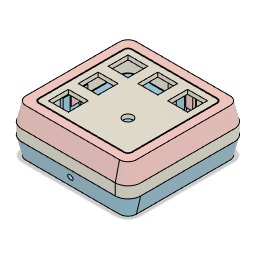
Pico_Macropad v37 (Autodesk Fusion 360 design; units mm, degrees)
Autodesk Fusion 360 part; units mm, degrees
note: some values were not read from the file. Set by a fixed rule: which sketch regions a step uses.
ref_plane "WorkPlane3" through (0, 25.4, 0) normal (0, 1, 0) x (0, 0, 1) in component "switchesPlate"
sketch "keycapsSwitches" plane through (0, 25.4, 0) normal (0, 1, 0) x (1, 0, 0) in component "switchesPlate"
  line L0 (-30.15, -30.15) -> (-12.05, -30.15) construction
  line L1 (-12.05, -30.15) -> (-12.05, -12.05) construction
  line L2 (-12.05, -12.05) -> (-30.15, -12.05) construction
  line L3 (-30.15, -12.05) -> (-30.15, -30.15) construction
  line L4 (-28.1, -28.1) -> (-14.1, -28.1)
  line L5 (-14.1, -28.1) -> (-14.1, -14.1)
  line L6 (-14.1, -14.1) -> (-28.1, -14.1)
  line L7 (-28.1, -14.1) -> (-28.1, -28.1)
  line L8 (-21.1, -12.05) -> (-21.1, -30.15) construction
  line L9 (-12.05, -21.1) -> (-30.15, -21.1) construction
  line L10 (-9.05, -12.05) -> (-9.05, -30.15) construction
  line L11 (7, -28.1) -> (7, -14.1)
  line L12 (-7, -28.1) -> (7, -28.1)
  line L13 (-7, -14.1) -> (-7, -28.1)
  line L14 (9.05, -21.1) -> (-9.05, -21.1) construction
  line L15 (7, -14.1) -> (-7, -14.1)
  line L16 (9.05, -12.05) -> (-9.05, -12.05) construction
  line L17 (0, -12.05) -> (0, -30.15) construction
  line L18 (-9.05, -30.15) -> (9.05, -30.15) construction
  line L19 (9.05, -30.15) -> (9.05, -12.05) construction
  line L20 (12.05, -12.05) -> (12.05, -30.15) construction
  line L21 (30.15, -21.1) -> (12.05, -21.1) construction
  line L22 (12.05, -30.15) -> (30.15, -30.15) construction
  line L23 (28.1, -14.1) -> (14.1, -14.1)
  line L24 (30.15, -12.05) -> (12.05, -12.05) construction
  line L25 (28.1, -28.1) -> (28.1, -14.1)
  line L26 (21.1, -12.05) -> (21.1, -30.15) construction
  line L27 (30.15, -30.15) -> (30.15, -12.05) construction
  line L28 (14.1, -14.1) -> (14.1, -28.1)
  line L29 (14.1, -28.1) -> (28.1, -28.1)
  line L30 (12.05, 9.05) -> (12.05, -9.05) construction
  line L31 (30.15, 0) -> (12.05, 0) construction
  line L32 (12.05, -9.05) -> (30.15, -9.05) construction
  line L33 (30.15, 9.05) -> (12.05, 9.05) construction
  line L34 (21.1, 9.05) -> (21.1, -9.05) construction
  line L35 (28.1, -7) -> (28.1, 7)
  line L36 (28.1, 7) -> (14.1, 7)
  line L37 (14.1, -7) -> (28.1, -7)
  line L38 (30.15, -9.05) -> (30.15, 9.05) construction
  line L39 (14.1, 7) -> (14.1, -7)
  line L40 (21.1, 30.15) -> (21.1, 12.05) construction
  line L41 (30.15, 12.05) -> (30.15, 30.15) construction
  line L42 (14.1, 14.1) -> (28.1, 14.1)
  line L43 (28.1, 28.1) -> (14.1, 28.1)
  line L44 (30.15, 21.1) -> (12.05, 21.1) construction
  line L45 (14.1, 28.1) -> (14.1, 14.1)
  line L46 (30.15, 30.15) -> (12.05, 30.15) construction
  line L47 (12.05, 30.15) -> (12.05, 12.05) construction
  line L48 (28.1, 14.1) -> (28.1, 28.1)
  line L49 (12.05, 12.05) -> (30.15, 12.05) construction
  line L50 (-33.15, 33.15) -> (33.15, 33.15) construction
  line L51 (33.15, 33.15) -> (33.15, -33.15) construction
  line L52 (33.15, -33.15) -> (-33.15, -33.15) construction
  line L53 (-33.15, -33.15) -> (-33.15, 33.15) construction
  dimension "d136" = 18.1
  dimension "d147" = 14
  dimension "d150" = 7
  dimension "d151" = 7
  dimension "d152" = 18.1
  dimension "d153" = 14
  dimension "d154" = 7
  dimension "d155" = 7
  dimension "d156" = 18.1
  dimension "d157" = 14
  dimension "d158" = 7
  dimension "d159" = 7
  dimension "d160" = 18.1
  dimension "d161" = 14
  dimension "d162" = 7
  dimension "d163" = 7
  dimension "d164" = 18.1
  dimension "d165" = 14
  dimension "d166" = 7
  dimension "d167" = 7
  dimension "d168" = 3
  dimension "d169" = 3
  dimension "d170" = 3
  dimension "d171" = 3
  dimension "d173" = 3
  dimension "d174" = 3
  dimension "d175" = 3
  dimension "d176" = 3
  constraint horizontal L0
  constraint vertical L1
  constraint horizontal L2
  constraint vertical L3
  constraint equal L1 L2
  constraint horizontal L4
  constraint vertical L5
  constraint horizontal L6
  constraint vertical L7
  constraint equal L4 L5
  constraint midpoint L2 L8.start
  constraint midpoint L0 L8.end
  constraint midpoint L1 L9.start
  constraint midpoint L3 L9.end
  constraint horizontal L18
  constraint vertical L19
  constraint horizontal L16
  constraint vertical L10
  constraint equal L16 L19
  constraint horizontal L12
  constraint vertical L11
  constraint horizontal L15
  constraint vertical L13
  constraint equal L11 L12
  constraint midpoint L17.start L16
  constraint midpoint L17.end L18
  constraint midpoint L14.start L19
  constraint midpoint L14.end L10
  constraint horizontal L22
  constraint vertical L27
  constraint horizontal L24
  constraint vertical L20
  constraint equal L24 L27
  constraint horizontal L29
  constraint vertical L25
  constraint horizontal L23
  constraint vertical L28
  constraint equal L25 L29
  constraint midpoint L26.start L24
  constraint midpoint L26.end L22
  constraint midpoint L21.start L27
  constraint midpoint L21.end L20
  constraint horizontal L32
  constraint vertical L38
  constraint horizontal L33
  constraint vertical L30
  constraint equal L33 L38
  constraint horizontal L37
  constraint vertical L35
  constraint horizontal L36
  constraint vertical L39
  constraint equal L35 L37
  constraint midpoint L34.start L33
  constraint midpoint L34.end L32
  constraint midpoint L31.start L38
  constraint midpoint L31.end L30
  constraint horizontal L49
  constraint vertical L41
  constraint horizontal L46
  constraint vertical L47
  constraint equal L41 L46
  constraint horizontal L42
  constraint vertical L48
  constraint horizontal L43
  constraint vertical L45
  constraint equal L42 L48
  constraint midpoint L40.start L46
  constraint midpoint L40.end L49
  constraint midpoint L44.start L41
  constraint midpoint L44.end L47
  constraint coincident L20 L30.end
  constraint coincident L30 L47.end
  constraint coincident origin L17
  constraint coincident L5.end L15
  constraint coincident L18 L20.end
  constraint coincident origin L31
  constraint horizontal L50
  constraint vertical L51
  constraint horizontal L52
  constraint vertical L53
  measures "d136" distance of L1.end L2.end
  measures "d147" distance of L4.end L5.end
  measures "d150" distance of L5.end L8
  measures "d151" distance of L4.end L9
  measures "d152" distance of L16.start L10.start
  measures "d153" distance of L11.start L11.end
  measures "d154" distance of L11.end L17
  measures "d155" distance of L11.start L14
  measures "d156" distance of L20.start L24.start
  measures "d157" distance of L23.start L25.start
  measures "d158" distance of L23.start L26
  measures "d159" distance of L25.start L21
  measures "d160" distance of L30.start L33.start
  measures "d161" distance of L35.end L35.start
  measures "d162" distance of L35.end L34
  measures "d163" distance of L35.start L31
  measures "d164" distance of L46.end L41.end
  measures "d165" distance of L43.start L42.end
  measures "d166" distance of L43.start L40
  measures "d167" distance of L42.end L44
  measures "d168" horizontal distance of L1.end L10.start
  measures "d169" distance of L16.start L20.start
  measures "d170" distance of L24.start L32.end
  measures "d171" distance of L33.start L41.start
  measures "d173" distance of L22.end L52
  measures "d174" distance of L41.end L51
  measures "d175" distance of L41.end L50
  measures "d176" distance of L3 L52.end
sketch "encoder" plane through (0, 25.4, 0) normal (0, 1, 0) x (1, 0, 0) in component "switchesPlate"
  line L0 (12.05, 30.15) -> (12.05, 12.05)
  line L1 (12.05, 9.05) -> (12.05, -9.05)
  line L2 (9.05, -12.05) -> (-9.05, -12.05)
  line L3 (-12.05, -12.05) -> (-30.15, -12.05)
  line L4 (-33.15, 33.15) -> (33.15, 33.15)
  line L5 (-33.15, -33.15) -> (-33.15, 33.15)
  line L6 (12.05, -12.05) -> (-33.15, 33.15) construction
  circle A0 centre (-10.55, 10.55) radius 3.5
  dimension "d177" = 7
  constraint coincident L4.start L5.end
  constraint coincident L2 L6.start
  constraint coincident L1 L6.start
  constraint midpoint L6 A0.centre
  measures "d177" diameter of A0
ref_plane "WorkPlane4" through (0, 22.4, 0) normal (0, 1, 0) x (0, 0, 1) in component "switchesPlate"
sketch "switchPlate" plane through (0, 22.4, 0) normal (0, 1, 0) x (1, 0, 0) in component "switchesPlate"
  line L0 (-36.15, 36.15) -> (36.15, 36.15)
  line L1 (36.15, 36.15) -> (36.15, -36.15)
  line L2 (36.15, -36.15) -> (-36.15, -36.15)
  line L3 (-36.15, -36.15) -> (-36.15, 36.15)
  line L4 (-33.15, 33.15) -> (33.15, 33.15)
  line L5 (33.15, 33.15) -> (33.15, -33.15)
  line L6 (33.15, -33.15) -> (-33.15, -33.15)
  line L7 (-33.15, -33.15) -> (-33.15, 33.15)
  line L8 (-33.15, 33.15) -> (33.15, 33.15)
  point P0 (33.15, -33.15)
  point P1 (-33.15, 33.15)
  point P2 (33.15, 33.15)
  point P3 (33.15, 33.15)
  dimension "d180" = 3
  dimension "d181" = 3
  dimension "d182" = 3
  dimension "d183" = 3
  constraint horizontal L0
  constraint vertical L1
  constraint horizontal L2
  constraint vertical L3
  constraint horizontal L4
  constraint vertical L5
  constraint horizontal L6
  constraint vertical L7
  constraint coincident P0 L5.end
  constraint coincident P1 L4.start
  measures "d180" horizontal distance of L0.end P3
  measures "d181" horizontal distance of L0.start L4.start
  measures "d182" vertical distance of L1.end P0
  measures "d183" vertical distance of L0.end P3
extrude "Extrude13" add sketch "switchPlate" along normal blind 1 contours L0 L1 L2 L3 | L4 L5 L6 L7 L8 makes body 1 in component "switchesPlate"
extrude "Extrude14" add sketch "switchPlate" along normal blind 3 contours L4 L5 L6 L7 L8 bodies 1 in component "switchesPlate"
fillet "Fillet4" radius 3 8 edges at (33.15, 24.4, 33.15) (36.15, 22.9, 36.15) (36.15, 22.9, -36.15) (33.15, 24.4, -33.15) (-33.15, 24.4, -33.15) (-36.15, 22.9, -36.15) (-36.15, 22.9, 36.15) (-33.15, 24.4, 33.15) on bodies 1 in component "switchesPlate"
sketch "loftIn1" plane through (0, 25.4, 0) normal (0, 1, 0) x (-1, 0, 0) in component "case"
  arc A0 (33.15, 30.15) -> (30.15, 33.15) centre (30.15, 30.15) ccw
  line L0 (30.15, 33.15) -> (-30.15, 33.15)
  arc A1 (-30.15, 33.15) -> (-33.15, 30.15) centre (-30.15, 30.15) ccw
  line L1 (-33.15, 30.15) -> (-33.15, -30.15)
  arc A2 (-33.15, -30.15) -> (-30.15, -33.15) centre (-30.15, -30.15) ccw
  line L2 (-30.15, -33.15) -> (30.15, -33.15)
  arc A3 (30.15, -33.15) -> (33.15, -30.15) centre (30.15, -30.15) ccw
  line L3 (33.15, -30.15) -> (33.15, 30.15)
  arc A4 (36.15, 33.15) -> (33.15, 36.15) centre (33.15, 33.15) ccw
  line L4 (-33.15, 36.15) -> (33.15, 36.15)
  line L5 (36.15, 33.15) -> (36.15, -33.15)
  arc A5 (33.15, -36.15) -> (36.15, -33.15) centre (33.15, -33.15) ccw
  line L6 (33.15, -36.15) -> (-33.15, -36.15)
  arc A6 (-36.15, -33.15) -> (-33.15, -36.15) centre (-33.15, -33.15) ccw
  line L7 (-36.15, -33.15) -> (-36.15, 33.15)
  arc A7 (-33.15, 36.15) -> (-36.15, 33.15) centre (-33.15, 33.15) ccw
  line L8 (33.15, -39.15) -> (-33.15, -39.15)
  arc A8 (-39.15, -33.15) -> (-33.15, -39.15) centre (-33.15, -33.15) ccw
  line L9 (-39.15, -33.15) -> (-39.15, 33.15)
  arc A9 (-33.15, 39.15) -> (-39.15, 33.15) centre (-33.15, 33.15) ccw
  line L10 (-33.15, 39.15) -> (33.15, 39.15)
  arc A10 (39.15, 33.15) -> (33.15, 39.15) centre (33.15, 33.15) ccw
  line L11 (39.15, 33.15) -> (39.15, -33.15)
  arc A11 (33.15, -39.15) -> (39.15, -33.15) centre (33.15, -33.15) ccw
  dimension "d190" = 3
ref_plane "WorkPlane4" through (0, 12.7, 0) normal (0, 1, 0) x (0, 0, 1) in component "case"
sketch "loftin2" plane through (0, 12.7, 0) normal (0, 1, 0) x (1, 0, 0) in component "case"
  arc A0 (33.15, -39.15) -> (39.15, -33.15) centre (33.15, -33.15) ccw
  line L0 (33.15, -39.15) -> (-33.15, -39.15)
  arc A1 (-39.15, -33.15) -> (-33.15, -39.15) centre (-33.15, -33.15) ccw
  line L1 (-39.15, -33.15) -> (-39.15, 33.15)
  arc A2 (-33.15, 39.15) -> (-39.15, 33.15) centre (-33.15, 33.15) ccw
  line L2 (-33.15, 39.15) -> (33.15, 39.15)
  arc A3 (39.15, 33.15) -> (33.15, 39.15) centre (33.15, 33.15) ccw
  line L3 (39.15, 33.15) -> (39.15, -33.15)
  arc A4 (-42.15, -33.15) -> (-33.15, -42.15) centre (-33.15, -33.15) ccw
  line L4 (33.15, -42.15) -> (-33.15, -42.15)
  arc A5 (33.15, -42.15) -> (42.15, -33.15) centre (33.15, -33.15) ccw
  line L5 (42.15, 33.15) -> (42.15, -33.15)
  arc A6 (42.15, 33.15) -> (33.15, 42.15) centre (33.15, 33.15) ccw
  line L6 (-33.15, 42.15) -> (33.15, 42.15)
  arc A7 (-33.15, 42.15) -> (-42.15, 33.15) centre (-33.15, 33.15) ccw
  line L7 (-42.15, -33.15) -> (-42.15, 33.15)
  dimension "d192" = 3
loft "Loft8" add profiles "loftin2" section 1 face at (11.05, 22.4, -12.05) section 2 contours A0 L0 A1 L1 A2 L2 A3 L3 separate body on bodies 1 makes body 2 in component "case"
loft "Loft9" add profiles "loftin2", "loftIn1" section 1 section 2 contours L8 A8 L9 A9 L10 A10 L11 A11 separate body makes body 3 in component "case"
combine "Combine9" operation cut target body 3 tool bodies 2 keep tools in component "case"
sketch "tooth" plane through (0, 0, 0) normal (0, 0, 1) x (1, 0, 0) in component "case"
  line L0 (39.15, 25.4) -> (-39.15, 25.4)
  line L1 (42.15, 12.7) -> (39.15, 12.7)
  line L2 (-39.15, 12.7) -> (-42.15, 12.7)
  line L3 (42.15, 12.7) -> (39.15, 25.4)
  line L4 (-42.15, 12.7) -> (-39.15, 25.4)
  line L5 (39.15, 12.7) -> (-39.15, 12.7)
  line L6 (36.15, 22.4) -> (-36.15, 22.4)
  line L7 (36.15, 22.4) -> (39.15, 12.7)
  line L8 (-36.15, 22.4) -> (-39.15, 12.7)
  line L9 (-39.15, 12.7) -> (-39.15, 4.7)
  line L10 (-39.15, 4.7) -> (-37.15, 4.7)
  line L11 (-37.15, 4.7) -> (-37.15, 19.1667)
  line L12 (-37.15, 19.1667) -> (-39.15, 12.7)
  dimension "d221" = 2
  dimension "d222" = 8
  constraint coincident L2.start L5.end
  constraint perpendicular L2 L9
  constraint perpendicular L9 L10
  constraint perpendicular L5 L11
  constraint coincident L8 L11.end
  constraint coincident L11.end L12.start
  measures "d221" distance of L9.end L10.end
  measures "d222" distance of L2.start L9.end
extrude "Extrude3" add sketch "tooth" along normal mid plane 6 contours L5 L8 L11 L12 | L5 L9 L10 L11 bodies 3 in component "case"
pattern_circular "C-Pattern1" count 2 over 360 about axis through (0, 1.75, 0) along (0, 1, 0) of "Extrude3" in component "case"
ref_plane "WorkPlane5" through (3.75, 0, 0) normal (1, 0, 0) x (0, 1, 0) in component "case"
sketch "doubletooth" plane through (3.75, 0, 0) normal (1, 0, 0) x (0, 0, -1) in component "case"
  line L0 (-42.15, 12.7) -> (42.15, 12.7)
  line L1 (-42.15, 12.7) -> (-39.15, 25.4)
  line L2 (-39.15, 25.4) -> (39.15, 25.4)
  line L3 (-3, 4.7) -> (3, 4.7)
  line L4 (3, 4.7) -> (3, 12.7)
  line L5 (-3, 12.7) -> (3, 12.7)
  line L6 (-3, 12.7) -> (-3, 4.7)
  line L7 (3, 12.7) -> (3, 19.1667)
  line L8 (3, 19.1667) -> (-3, 19.1667)
  line L9 (-3, 19.1667) -> (-3, 12.7)
  line L10 (-39.15, 12.7) -> (-3, 12.7)
  line L11 (-39.15, 12.7) -> (-36.15, 22.4)
  line L12 (-36.15, 22.4) -> (36.15, 22.4)
  line L13 (-3, 12.7) -> (-39.15, 12.7)
  line L14 (-3, 12.7) -> (-3, 19.1667)
  line L15 (-3, 19.1667) -> (3, 19.1667)
  line L16 (3, 19.1667) -> (3, 12.7)
  line L17 (3, 12.7) -> (39.15, 12.7)
  line L18 (-37.15, 19.1667) -> (-37.15, 4.7)
  line L19 (-37.15, 4.7) -> (-39.15, 4.7)
  line L20 (-39.15, 4.7) -> (-39.15, 12.7)
  line L21 (-39.15, 25.4) -> (-42.15, 12.7)
  line L22 (-36.15, 22.4) -> (-39.15, 12.7)
  dimension "d230" = 2
  constraint perpendicular L10 L18
  constraint coincident L10.start L11.start
  constraint coincident L3 L19.end
  constraint perpendicular L18 L19
  constraint perpendicular L19 L20
  constraint coincident L11.end L12.start
  constraint coincident L11 L18.start
  measures "d230" distance of L18.end L19.end
extrude "Extrude6" add sketch "doubletooth" along normal blind 5 contours L0 L10 L11 L13 L18 L22 | L0 L10 L13 L18 L19 L20 bodies 3 in component "case"
mirror "Mirror4" about plane through (0, 0, 0) normal (1, 0, 0) of "Extrude6" in component "case"
mirror "Mirror5" about plane through (0, 0, 0) normal (0, 0, 1) of "Extrude6", "Mirror4" in component "case"
sketch "bandSketch" plane through (0, 12.7, 0) normal (0, -1, 0) x (1, 0, 0) in component "case"
  line L0 (-39.15, -3) -> (-39.15, 3)
  spline S0 degree 3 poles (33.15, 42.15) (34.1498, 42.15) (35.3159, 41.9726) (36.4656, 41.517) (37.3209, 41.1781) (38.1632, 40.6875) (38.9102, 40.0652) (40.0083, 39.1505) (40.8849, 37.9488) (41.422, 36.696) (41.9461, 35.4734) (42.15, 34.2167) (42.15, 33.15) (42.15, 11.05) (42.15, -11.05) (42.15, -33.15) (42.15, -34.1498) (41.9726, -35.3159) (41.517, -36.4656) (41.1781, -37.3209) (40.6875, -38.1632) (40.0652, -38.9102) (39.1505, -40.0083) (37.9488, -40.8849) (36.696, -41.422) (35.4734, -41.9461) (34.2167, -42.15) (33.15, -42.15) (11.05, -42.15) (-11.05, -42.15) (-33.15, -42.15) (-34.1498, -42.15) (-35.3159, -41.9726) (-36.4656, -41.517) (-37.3209, -41.1781) (-38.1632, -40.6875) (-38.9102, -40.0652) (-40.0083, -39.1505) (-40.8849, -37.9488) (-41.422, -36.696) (-41.9461, -35.4734) (-42.15, -34.2167) (-42.15, -33.15) (-42.15, -11.05) (-42.15, 11.05) (-42.15, 33.15) (-42.15, 34.1498) (-41.9726, 35.3159) (-41.517, 36.4656) (-41.1781, 37.3209) (-40.6875, 38.1632) (-40.0652, 38.9102) (-39.1505, 40.0083) (-37.9488, 40.8849) (-36.696, 41.422) (-35.4734, 41.9461) (-34.2167, 42.15) (-33.15, 42.15) (-11.05, 42.15) (11.05, 42.15) (33.15, 42.15) knots 0 0 0 0 0.009612 0.009612 0.009612 0.016762 0.016762 0.016762 0.027271 0.027271 0.027271 0.037527 0.037527 0.037527 0.25 0.25 0.25 0.259612 0.259612 0.259612 0.266762 0.266762 0.266762 0.277271 0.277271 0.277271 0.287527 0.287527 0.287527 0.5 0.5 0.5 0.509612 0.509612 0.509612 0.516762 0.516762 0.516762 0.527271 0.527271 0.527271 0.537527 0.537527 0.537527 0.75 0.75 0.75 0.759612 0.759612 0.759612 0.766762 0.766762 0.766762 0.777271 0.777271 0.777271 0.787527 0.787527 0.787527 1 1 1 1
  line L1 (-33.15, 39.15) -> (-8.75, 39.15)
  line L2 (39.15, 3) -> (39.15, -3)
  line L3 (-8.75, 39.15) -> (-3.75, 39.15)
  line L4 (-3.75, 39.15) -> (3.75, 39.15)
  line L5 (3.75, 39.15) -> (8.75, 39.15)
  spline S1 degree 3 poles (8.75, 39.15) (16.8833, 39.15) (25.0167, 39.15) (33.15, 39.15) (33.7471, 39.15) (34.5104, 39.053) (35.2899, 38.7554) (35.8698, 38.534) (36.4549, 38.2028) (36.9737, 37.7738) (37.7361, 37.1433) (38.3397, 36.2995) (38.6931, 35.4465) (39.038, 34.6141) (39.15, 33.787) (39.15, 33.15) (39.15, 23.1) (39.15, 13.05) (39.15, 3) knots 0.14292 0.14292 0.14292 0.14292 0.226147 0.226147 0.226147 0.232257 0.232257 0.232257 0.236802 0.236802 0.236802 0.243482 0.243482 0.243482 0.25 0.25 0.25 0.352841 0.352841 0.352841 0.352841
  spline S2 degree 3 poles (39.15, -3) (39.15, -13.05) (39.15, -23.1) (39.15, -33.15) (39.15, -33.7471) (39.053, -34.5104) (38.7554, -35.2899) (38.534, -35.8698) (38.2028, -36.4549) (37.7738, -36.9737) (37.1433, -37.7361) (36.2995, -38.3397) (35.4465, -38.6931) (34.6141, -39.038) (33.787, -39.15) (33.15, -39.15) (25.0167, -39.15) (16.8833, -39.15) (8.75, -39.15) knots 0.373307 0.373307 0.373307 0.373307 0.476147 0.476147 0.476147 0.482257 0.482257 0.482257 0.486802 0.486802 0.486802 0.493482 0.493482 0.493482 0.5 0.5 0.5 0.583228 0.583228 0.583228 0.583228
  line L6 (8.75, -39.15) -> (3.75, -39.15)
  line L7 (3.75, -39.15) -> (-3.75, -39.15)
  line L8 (-3.75, -39.15) -> (-8.75, -39.15)
  spline S3 degree 3 poles (-8.75, -39.15) (-16.8833, -39.15) (-25.0167, -39.15) (-33.15, -39.15) (-33.7471, -39.15) (-34.5104, -39.053) (-35.2899, -38.7554) (-35.8698, -38.534) (-36.4549, -38.2028) (-36.9737, -37.7738) (-37.7361, -37.1433) (-38.3397, -36.2995) (-38.6931, -35.4465) (-39.038, -34.6141) (-39.15, -33.787) (-39.15, -33.15) (-39.15, -23.1) (-39.15, -13.05) (-39.15, -3) knots 0.64292 0.64292 0.64292 0.64292 0.726147 0.726147 0.726147 0.732257 0.732257 0.732257 0.736802 0.736802 0.736802 0.743482 0.743482 0.743482 0.75 0.75 0.75 0.852841 0.852841 0.852841 0.852841
  spline S4 degree 3 poles (-39.15, 3) (-39.15, 13.05) (-39.15, 23.1) (-39.15, 33.15) (-39.15, 33.7471) (-39.053, 34.5104) (-38.7554, 35.2899) (-38.534, 35.8698) (-38.2028, 36.4549) (-37.7738, 36.9737) (-37.1433, 37.7361) (-36.2995, 38.3397) (-35.4465, 38.6931) (-34.6141, 39.038) (-33.787, 39.15) (-33.15, 39.15) knots 0.873307 0.873307 0.873307 0.873307 0.976147 0.976147 0.976147 0.982257 0.982257 0.982257 0.986802 0.986802 0.986802 0.993482 0.993482 0.993482 1 1 1 1
extrude "Extrude4" add sketch "bandSketch" along normal up to surface (8 mm away) separate body makes body 4 in component "case"
copy_body "CopyPasteBodies1" bodies 3 makes body 5
move_body "Move1" bodies 5 to x (0, 0, 1) y (0, -1, 0) z (1, 0, 0) at (0, 22.4, 0)
copy_body "CutPasteBodies4" bodies 5 removing the originals makes body 6 in component "case"
combine "Combine10" operation cut target body 3 tool bodies 1 keep tools in component "case"
extrude "Extrude15" cut sketch "encoder" sketch "keycapsSwitches" along normal up to surface of sketch 2 end surface through (0, 22.4, 0) normal (0, -1, 0) offset 0 bodies 1 in component "switchesPlate"
sketch "tolerancePlateTop" plane through (0, 25.4, 0) normal (0, 1, 0) x (-1, 0, 0) in component "switchesPlate"
  line L0 (-14.1, 28.1) -> (-14.1, 14.1)
  line L1 (-14.1, 14.1) -> (-28.1, 14.1)
  line L2 (-28.1, 14.1) -> (-28.1, 28.1)
  line L3 (-28.1, 28.1) -> (-14.1, 28.1)
  line L4 (-14.1, -7) -> (-28.1, -7)
  line L5 (-28.1, -7) -> (-28.1, 7)
  line L6 (-28.1, 7) -> (-14.1, 7)
  line L7 (-14.1, 7) -> (-14.1, -7)
  circle A0 centre (10.55, -10.55) radius 3.5
  line L8 (-7, 14.1) -> (-7, 28.1)
  line L9 (-7, 28.1) -> (7, 28.1)
  line L10 (7, 28.1) -> (7, 14.1)
  line L11 (7, 14.1) -> (-7, 14.1)
  line L12 (-28.1, -14.1) -> (-14.1, -14.1)
  line L13 (-14.1, -14.1) -> (-14.1, -28.1)
  line L14 (-14.1, -28.1) -> (-28.1, -28.1)
  line L15 (-28.1, -28.1) -> (-28.1, -14.1)
  line L16 (28.1, 14.1) -> (14.1, 14.1)
  line L17 (14.1, 14.1) -> (14.1, 28.1)
  line L18 (14.1, 28.1) -> (28.1, 28.1)
  line L19 (28.1, 28.1) -> (28.1, 14.1)
  arc A1 (33.15, 30.15) -> (30.15, 33.15) centre (30.15, 30.15) ccw
  line L20 (30.15, 33.15) -> (-30.15, 33.15)
  arc A2 (-30.15, 33.15) -> (-33.15, 30.15) centre (-30.15, 30.15) ccw
  line L21 (-33.15, 30.15) -> (-33.15, -30.15)
  arc A3 (-33.15, -30.15) -> (-30.15, -33.15) centre (-30.15, -30.15) ccw
  line L22 (-30.15, -33.15) -> (30.15, -33.15)
  arc A4 (30.15, -33.15) -> (33.15, -30.15) centre (30.15, -30.15) ccw
  line L23 (33.15, -30.15) -> (33.15, 30.15)
  line L24 (30.15, 32.65) -> (-30.15, 32.65)
  arc A5 (-30.15, 32.65) -> (-32.65, 30.15) centre (-30.15, 30.15) ccw
  line L25 (-32.65, 30.15) -> (-32.65, -30.15)
  arc A6 (-32.65, -30.15) -> (-30.15, -32.65) centre (-30.15, -30.15) ccw
  line L26 (-30.15, -32.65) -> (30.15, -32.65)
  arc A7 (30.15, -32.65) -> (32.65, -30.15) centre (30.15, -30.15) ccw
  line L27 (32.65, -30.15) -> (32.65, 30.15)
  arc A8 (32.65, 30.15) -> (30.15, 32.65) centre (30.15, 30.15) ccw
  dimension "d208" = -0.5
extrude "Extrude16" cut sketch "tolerancePlateTop" against normal up to surface (2 mm away) contours A1 L20 A2 L21 A3 L22 A4 L23 bodies 1 in component "switchesPlate"
sketch "tolerancePlateInner" plane through (0, 23.4, 0) normal (0, 1, 0) x (-1, 0, 0) in component "switchesPlate"
  arc A0 (36.15, 33.15) -> (33.15, 36.15) centre (33.15, 33.15) ccw
  line L0 (33.15, 36.15) -> (-33.15, 36.15)
  arc A1 (-33.15, 36.15) -> (-36.15, 33.15) centre (-33.15, 33.15) ccw
  line L1 (-36.15, 33.15) -> (-36.15, -33.15)
  arc A2 (-36.15, -33.15) -> (-33.15, -36.15) centre (-33.15, -33.15) ccw
  line L2 (-33.15, -36.15) -> (33.15, -36.15)
  arc A3 (33.15, -36.15) -> (36.15, -33.15) centre (33.15, -33.15) ccw
  line L3 (36.15, -33.15) -> (36.15, 33.15)
  arc A4 (33.15, -35.65) -> (35.65, -33.15) centre (33.15, -33.15) ccw
  line L4 (35.65, -33.15) -> (35.65, 33.15)
  arc A5 (35.65, 33.15) -> (33.15, 35.65) centre (33.15, 33.15) ccw
  line L5 (33.15, 35.65) -> (-33.15, 35.65)
  arc A6 (-33.15, 35.65) -> (-35.65, 33.15) centre (-33.15, 33.15) ccw
  line L6 (-35.65, 33.15) -> (-35.65, -33.15)
  arc A7 (-35.65, -33.15) -> (-33.15, -35.65) centre (-33.15, -33.15) ccw
  line L7 (-33.15, -35.65) -> (33.15, -35.65)
  line L8 (32.65, 30.15) -> (32.65, -30.15)
  arc A8 (30.15, -32.65) -> (32.65, -30.15) centre (30.15, -30.15) ccw
  line L9 (30.15, -32.65) -> (-30.15, -32.65)
  arc A9 (-32.65, -30.15) -> (-30.15, -32.65) centre (-30.15, -30.15) ccw
  line L10 (-32.65, -30.15) -> (-32.65, 30.15)
  arc A10 (-30.15, 32.65) -> (-32.65, 30.15) centre (-30.15, 30.15) ccw
  line L11 (-30.15, 32.65) -> (30.15, 32.65)
  arc A11 (32.65, 30.15) -> (30.15, 32.65) centre (30.15, 30.15) ccw
  dimension "d211" = -0.5
extrude "Extrude17" cut sketch "tolerancePlateInner" against normal up to surface (1 mm away) contours A0 L0 A1 L1 A2 L2 A3 L3 bodies 1 in component "switchesPlate"
move_body "Move5" bodies 6 to x (1, 0, 0) y (0, 1, 0) z (0, 0, 1) at (0, -5, 0) in component "case"
sketch "USBhole" plane through (0, 0, 0) normal (0, 0, 1) x (1, 0, 0) in component "case"
  line L0 (-3, 12.7) -> (3, 12.7)
  line L1 (3, 4.7) -> (3, 12.7)
  line L2 (-39.15, -8) -> (39.15, -8)
  line L3 (-42.15, 4.7) -> (-39.15, 4.7)
  line L4 (-37.15, 4.7) -> (-3, 4.7)
  line L5 (3, 4.7) -> (37.15, 4.7)
  line L6 (39.15, 4.7) -> (42.15, 4.7)
  line L7 (-42.15, 4.7) -> (-39.15, -8)
  line L8 (42.15, 4.7) -> (39.15, -8)
  circle A0 centre (0, -1.1) radius 1.9
  line L9 (0, 1.75) -> (0, 22.5)
  line L10 (-1.9, 0.8) -> (1.9, 0.8) construction
  line L11 (1.9, 0.8) -> (1.9, -3) construction
  line L12 (1.9, -3) -> (-1.9, -3) construction
  line L13 (-1.9, -3) -> (-1.9, 0.8) construction
  line L14 (-39.15, 4.7) -> (-39.15, 12.7)
  line L15 (-37.15, 12.7) -> (-37.15, 4.7)
  line L16 (-39.15, 12.7) -> (-37.15, 12.7)
  line L17 (39.15, 4.7) -> (39.15, 12.7)
  line L18 (37.15, 12.7) -> (37.15, 4.7)
  line L19 (39.15, 12.7) -> (37.15, 12.7)
  line L20 (-3, 12.7) -> (-3, 4.7)
  line L21 (36.15, -5) -> (-36.15, -5)
  dimension "d216" = 3.8
  dimension "d231" = 2
  constraint horizontal L10
  constraint vertical L11
  constraint horizontal L12
  constraint vertical L13
  constraint tangent A0 L12
  constraint tangent A0 L11
  constraint tangent A0 L10
  constraint tangent A0 L13
  constraint coincident A0.centre L9
  measures "d216" diameter of A0
  measures "d231" distance of L12.end L21
extrude "Extrude7" cut sketch "USBhole" along normal blind 45 contours A0 bodies 6 in component "case"
move_body "Move4" bodies 1 to x (-1, 0, 0) y (0, 1, 0) z (0, 0, -1) at (0, 0, 0) in component "switchesPlate"
sketch "picoStandoffs" plane through (0, -9.8609, 0) normal (0, 1, 0) x (-1, 0, 0) in component "picoHolder"
  spline S0 degree 3 poles (-76.4563, -33.0811) (-76.4563, -18.1883) (-76.4563, 18.3262) (-76.4563, 33.2189) (-76.4563, 33.6213) (-76.3743, 34.0235) (-76.2168, 34.3937) (-76.0996, 34.6691) (-75.9409, 34.9268) (-75.7477, 35.1554) (-75.4638, 35.4913) (-75.1049, 35.7637) (-74.705, 35.9467) (-74.3146, 36.1254) (-73.8856, 36.2189) (-73.4563, 36.2189) (-58.5636, 36.2189) (-22.0491, 36.2189) (-7.1563, 36.2189) (-6.754, 36.2189) (-6.3518, 36.1369) (-5.9816, 35.9794) (-5.7062, 35.8622) (-5.4485, 35.7035) (-5.2199, 35.5103) (-4.8839, 35.2264) (-4.6116, 34.8675) (-4.4285, 34.4676) (-4.2499, 34.0772) (-4.1563, 33.6482) (-4.1563, 33.2189) (-4.1563, 18.3262) (-4.1563, -18.1883) (-4.1563, -33.0811) (-4.1563, -33.4834) (-4.2384, -33.8856) (-4.3959, -34.2558) (-4.5131, -34.5312) (-4.6718, -34.7889) (-4.865, -35.0175) (-5.1489, -35.3535) (-5.5077, -35.6258) (-5.9077, -35.8089) (-6.298, -35.9875) (-6.7271, -36.0811) (-7.1563, -36.0811) (-22.0491, -36.0811) (-58.5636, -36.0811) (-73.4563, -36.0811) (-73.8587, -36.0811) (-74.2609, -35.999) (-74.6311, -35.8415) (-74.9065, -35.7243) (-75.1642, -35.5656) (-75.3928, -35.3724) (-75.7287, -35.0885) (-76.0011, -34.7297) (-76.1841, -34.3297) (-76.3628, -33.9394) (-76.4563, -33.5103) (-76.4563, -33.0811) knots 0 0 0 0 0.226147 0.226147 0.226147 0.232257 0.232257 0.232257 0.236802 0.236802 0.236802 0.243482 0.243482 0.243482 0.25 0.25 0.25 0.476147 0.476147 0.476147 0.482257 0.482257 0.482257 0.486802 0.486802 0.486802 0.493482 0.493482 0.493482 0.5 0.5 0.5 0.726147 0.726147 0.726147 0.732257 0.732257 0.732257 0.736802 0.736802 0.736802 0.743482 0.743482 0.743482 0.75 0.75 0.75 0.976147 0.976147 0.976147 0.982257 0.982257 0.982257 0.986802 0.986802 0.986802 0.993482 0.993482 0.993482 1 1 1 1
  line L0 (-40.3063, 0.0689) -> (-40.3063, 36.2189) construction
  line L1 (-40.3063, 0.0689) -> (-40.3063, -36.0811) construction
  line L2 (-29.8063, 25.5689) -> (-50.8063, 25.5689) construction
  line L3 (-50.8063, 25.5689) -> (-50.8063, -25.4311) construction
  line L4 (-50.8063, -25.4311) -> (-29.8063, -25.4311) construction
  line L5 (-29.8063, -25.4311) -> (-29.8063, 25.5689) construction
  line L6 (-44.8063, -23.4311) -> (-48.8063, -23.4311)
  line L7 (-48.8063, -23.4311) -> (-48.8063, -19.4311)
  line L8 (-48.8063, -19.4311) -> (-52.8063, -19.4311)
  line L9 (-52.8063, -19.4311) -> (-52.8063, -27.4311)
  line L10 (-52.8063, -27.4311) -> (-44.8063, -27.4311)
  line L11 (-44.8063, -27.4311) -> (-44.8063, -23.4311)
  line L12 (-44.8063, -25.9311) -> (-51.3063, -25.9311)
  line L13 (-51.3063, -25.9311) -> (-51.3063, -19.4311)
  line L14 (-29.8063, 0.0689) -> (-50.8063, 0.0689) construction
  line L15 (-35.8063, -25.9311) -> (-29.3063, -25.9311)
  line L16 (-29.3063, -25.9311) -> (-29.3063, -19.4311)
  line L17 (-31.8063, -19.4311) -> (-27.8063, -19.4311)
  line L18 (-27.8063, -19.4311) -> (-27.8063, -27.4311)
  line L19 (-27.8063, -27.4311) -> (-35.8063, -27.4311)
  line L20 (-35.8063, -27.4311) -> (-35.8063, -23.4311)
  line L21 (-31.8063, -23.4311) -> (-31.8063, -19.4311)
  line L22 (-35.8063, -23.4311) -> (-31.8063, -23.4311)
  line L23 (-35.8063, 23.5689) -> (-31.8063, 23.5689)
  line L24 (-31.8063, 23.5689) -> (-31.8063, 19.5689)
  line L25 (-31.8063, 19.5689) -> (-27.8063, 19.5689)
  line L26 (-27.8063, 19.5689) -> (-27.8063, 27.5689)
  line L27 (-27.8063, 27.5689) -> (-35.8063, 27.5689)
  line L28 (-35.8063, 27.5689) -> (-35.8063, 23.5689)
  line L29 (-29.3063, 26.0689) -> (-29.3063, 19.5689)
  line L30 (-35.8063, 26.0689) -> (-29.3063, 26.0689)
  line L31 (-44.8063, 23.5689) -> (-48.8063, 23.5689)
  line L32 (-48.8063, 23.5689) -> (-48.8063, 19.5689)
  line L33 (-48.8063, 19.5689) -> (-52.8063, 19.5689)
  line L34 (-52.8063, 19.5689) -> (-52.8063, 27.5689)
  line L35 (-44.8063, 27.5689) -> (-44.8063, 23.5689)
  line L36 (-51.3063, 26.0689) -> (-51.3063, 19.5689)
  line L37 (-44.8063, 26.0689) -> (-51.3063, 26.0689)
  line L38 (-52.8063, 27.5689) -> (-44.8063, 27.5689)
  point P0 (-40.3063, 0.0689)
  dimension "d238" = 51
  dimension "d245" = 21
  dimension "d246" = 25.5
  dimension "d247" = 10.5
  dimension "d248" = 2
  dimension "d249" = 2
  dimension "d250" = 4
  dimension "d251" = 4
  dimension "d252" = 0.5
  dimension "d253" = 0.5
  constraint coincident P0 L0.start
  constraint coincident S0 L0.end
  constraint vertical L0
  constraint coincident S0 L1.end
  constraint coincident L0 L1.end
  constraint horizontal L2
  constraint vertical L3
  constraint horizontal L4
  constraint vertical L5
  constraint horizontal L6
  constraint perpendicular L6 L7
  constraint perpendicular L3 L8
  constraint perpendicular L6 L9
  constraint perpendicular L3 L10
  constraint perpendicular L4 L11
  constraint equal L6 L8
  constraint equal L7 L8
  constraint horizontal L12
  constraint coincident L8 L13.end
  constraint perpendicular L8 L13
  constraint coincident L11 L12.start
  constraint midpoint L5 L14.start
  constraint midpoint L3 L14.end
  constraint symmetric L1 L6.start L20.end
  constraint symmetric L1 L6.end L21.start
  constraint symmetric L1 L7.end L17.start
  constraint symmetric L1 L8.end L17.end
  constraint symmetric L1 L9.end L18.end
  constraint symmetric L1 L10.end L19.end
  constraint symmetric L1 L12.start L15.start
  constraint symmetric L1 L12.end L15.end
  constraint symmetric L1 L13.end L16.end
  constraint symmetric L6.start L14 L31.start
  constraint symmetric L6.end L14 L31.end
  constraint symmetric L7.end L14 L32.end
  constraint symmetric L8.end L14 L33.end
  constraint symmetric L9.end L14 L34.end
  constraint symmetric L10.end L14 L35.start
  constraint symmetric L12.start L14 L37.start
  constraint symmetric L12.end L14 L36.start
  constraint symmetric L13.end L14 L36.end
  constraint symmetric L14 L15.start L30.start
  constraint symmetric L14 L15.end L29.start
  constraint symmetric L14 L16.end L29.end
  constraint symmetric L14 L17.start L24.end
  constraint symmetric L14 L17.end L25.end
  constraint symmetric L14 L18.end L26.end
  constraint symmetric L14 L19.end L27.end
  constraint symmetric L14 L20.end L23.start
  constraint symmetric L14 L21.start L23.end
  measures "d238" distance of L2.start L4.end
  measures "d245" distance of L3.end L4.end
  measures "d246" distance of P0 L4
  measures "d247" distance of L1 L3.end
  measures "d248" distance of L4 L6
  measures "d249" distance of L3 L7.end
  measures "d250" distance of L6.start L10.end
  measures "d251" distance of L7.end L8.end
  measures "d252" distance of L4 L12.start
  measures "d253" distance of L3 L13.end
extrude "Extrude10" add sketch "picoStandoffs" along normal blind 4 contours L8 L9 L10 L11 L12 L13 | L15 L16 L17 L18 L19 L20 | L25 L26 L27 L28 L29 L30 | L33 L34 L35 L36 L37 L38 sketch seen with x (1, 0, 0) y (0, 1, 0) z (0, 0, 1) at (-40.3063, 4.8609, -0.0689) bodies 6 in component "case"
extrude "Extrude11" add sketch "picoStandoffs" along normal blind 2 contours L6 L7 L8 L11 L12 L13 | L15 L16 L17 L20 L21 L22 | L23 L24 L25 L28 L29 L30 | L31 L32 L33 L35 L36 L37 sketch seen with x (1, 0, 0) y (0, 1, 0) z (0, 0, 1) at (-40.3063, 4.8609, -0.0689) bodies 6 in component "case"
fillet "Fillet1" radius 2 4 edges at (12.5, -3, 27.5) (-12.5, -3, 27.5) (-12.5, -3, -27.5) (12.5, -3, -27.5) on bodies 6 in component "case"
sketch "Sketch20" plane through (0, 12.7, 0) normal (0, 1, 0) x (-1, 0, 0) in component "case"
  line L0 (39.15, 3) -> (39.15, -3)
  spline S0 degree 3 poles (8.75, -39.15) (16.8833, -39.15) (25.0167, -39.15) (33.15, -39.15) (33.7471, -39.15) (34.5104, -39.053) (35.2899, -38.7554) (35.8698, -38.534) (36.4549, -38.2028) (36.9737, -37.7738) (37.7361, -37.1433) (38.3397, -36.2995) (38.6931, -35.4465) (39.038, -34.6141) (39.15, -33.787) (39.15, -33.15) (39.15, -23.1) (39.15, -13.05) (39.15, -3) knots 0.64292 0.64292 0.64292 0.64292 0.726147 0.726147 0.726147 0.732257 0.732257 0.732257 0.736802 0.736802 0.736802 0.743482 0.743482 0.743482 0.75 0.75 0.75 0.852841 0.852841 0.852841 0.852841
  line L1 (8.75, -39.15) -> (-8.75, -39.15)
  spline S1 degree 3 poles (-39.15, -3) (-39.15, -13.05) (-39.15, -23.1) (-39.15, -33.15) (-39.15, -33.7471) (-39.053, -34.5104) (-38.7554, -35.2899) (-38.534, -35.8698) (-38.2028, -36.4549) (-37.7738, -36.9737) (-37.1433, -37.7361) (-36.2995, -38.3397) (-35.4465, -38.6931) (-34.6141, -39.038) (-33.787, -39.15) (-33.15, -39.15) (-25.0167, -39.15) (-16.8833, -39.15) (-8.75, -39.15) knots 0.373307 0.373307 0.373307 0.373307 0.476147 0.476147 0.476147 0.482257 0.482257 0.482257 0.486802 0.486802 0.486802 0.493482 0.493482 0.493482 0.5 0.5 0.5 0.583228 0.583228 0.583228 0.583228
  line L2 (-39.15, -3) -> (-39.15, 3)
  spline S2 degree 3 poles (-8.75, 39.15) (-16.8833, 39.15) (-25.0167, 39.15) (-33.15, 39.15) (-33.7471, 39.15) (-34.5104, 39.053) (-35.2899, 38.7554) (-35.8698, 38.534) (-36.4549, 38.2028) (-36.9737, 37.7738) (-37.7361, 37.1433) (-38.3397, 36.2995) (-38.6931, 35.4465) (-39.038, 34.6141) (-39.15, 33.787) (-39.15, 33.15) (-39.15, 23.1) (-39.15, 13.05) (-39.15, 3) knots 0.14292 0.14292 0.14292 0.14292 0.226147 0.226147 0.226147 0.232257 0.232257 0.232257 0.236802 0.236802 0.236802 0.243482 0.243482 0.243482 0.25 0.25 0.25 0.352841 0.352841 0.352841 0.352841
  line L3 (-8.75, 39.15) -> (33.15, 39.15)
  spline S3 degree 3 poles (39.15, 3) (39.15, 13.05) (39.15, 23.1) (39.15, 33.15) (39.15, 33.7471) (39.053, 34.5104) (38.7554, 35.2899) (38.534, 35.8698) (38.2028, 36.4549) (37.7738, 36.9737) (37.1433, 37.7361) (36.2995, 38.3397) (35.4465, 38.6931) (34.6141, 39.038) (33.787, 39.15) (33.15, 39.15) knots 0.873307 0.873307 0.873307 0.873307 0.976147 0.976147 0.976147 0.982257 0.982257 0.982257 0.986802 0.986802 0.986802 0.993482 0.993482 0.993482 1 1 1 1
  spline S4 degree 3 poles (-33.15, 42.15) (-34.1498, 42.15) (-35.3159, 41.9726) (-36.4656, 41.517) (-37.3209, 41.1781) (-38.1632, 40.6875) (-38.9102, 40.0652) (-40.0083, 39.1505) (-40.8849, 37.9488) (-41.422, 36.696) (-41.9461, 35.4734) (-42.15, 34.2167) (-42.15, 33.15) (-42.15, 11.05) (-42.15, -11.05) (-42.15, -33.15) (-42.15, -34.1498) (-41.9726, -35.3159) (-41.517, -36.4656) (-41.1781, -37.3209) (-40.6875, -38.1632) (-40.0652, -38.9102) (-39.1505, -40.0083) (-37.9488, -40.8849) (-36.696, -41.422) (-35.4735, -41.9461) (-34.2167, -42.15) (-33.15, -42.15) (-11.05, -42.15) (11.05, -42.15) (33.15, -42.15) (34.1498, -42.15) (35.3159, -41.9726) (36.4656, -41.517) (37.3209, -41.1781) (38.1632, -40.6875) (38.9102, -40.0652) (40.0083, -39.1505) (40.8849, -37.9488) (41.422, -36.696) (41.9461, -35.4734) (42.15, -34.2167) (42.15, -33.15) (42.15, -11.05) (42.15, 11.05) (42.15, 33.15) (42.15, 34.1498) (41.9726, 35.3159) (41.517, 36.4656) (41.1781, 37.3209) (40.6875, 38.1632) (40.0652, 38.9102) (39.1505, 40.0083) (37.9488, 40.8849) (36.696, 41.422) (35.4734, 41.9461) (34.2167, 42.15) (33.15, 42.15) (11.05, 42.15) (-11.05, 42.15) (-33.15, 42.15) knots 0 0 0 0 0.009612 0.009612 0.009612 0.016762 0.016762 0.016762 0.027271 0.027271 0.027271 0.037527 0.037527 0.037527 0.25 0.25 0.25 0.259612 0.259612 0.259612 0.266762 0.266762 0.266762 0.277271 0.277271 0.277271 0.287527 0.287527 0.287527 0.5 0.5 0.5 0.509612 0.509612 0.509612 0.516762 0.516762 0.516762 0.527271 0.527271 0.527271 0.537527 0.537527 0.537527 0.75 0.75 0.75 0.759612 0.759612 0.759612 0.766762 0.766762 0.766762 0.777271 0.777271 0.777271 0.787527 0.787527 0.787527 1 1 1 1
  line L4 (8.75, -39.65) -> (-8.75, -39.65)
  spline S5 degree 3 poles (-39.65, -3) (-39.65, -13.05) (-39.65, -23.1) (-39.65, -33.15) (-39.65, -33.8012) (-39.546, -34.6209) (-39.2225, -35.4683) (-38.9819, -36.0987) (-38.6252, -36.7287) (-38.1591, -37.2923) (-37.4716, -38.1237) (-36.5691, -38.7692) (-35.6379, -39.155) (-34.7327, -39.5301) (-33.8456, -39.65) (-33.15, -39.65) (-25.0167, -39.65) (-16.8833, -39.65) (-8.75, -39.65) knots 0.373307 0.373307 0.373307 0.373307 0.476147 0.476147 0.476147 0.482257 0.482257 0.482257 0.486802 0.486802 0.486802 0.493482 0.493482 0.493482 0.5 0.5 0.5 0.583228 0.583228 0.583228 0.583228
  line L5 (-39.65, -3) -> (-39.65, 3)
  spline S6 degree 3 poles (-8.75, 39.65) (-16.8833, 39.65) (-25.0167, 39.65) (-33.15, 39.65) (-33.8012, 39.65) (-34.6209, 39.546) (-35.4683, 39.2225) (-36.0987, 38.9819) (-36.7287, 38.6252) (-37.2923, 38.1591) (-38.1237, 37.4716) (-38.7692, 36.5691) (-39.155, 35.6379) (-39.5301, 34.7327) (-39.65, 33.8456) (-39.65, 33.15) (-39.65, 23.1) (-39.65, 13.05) (-39.65, 3) knots 0.14292 0.14292 0.14292 0.14292 0.226147 0.226147 0.226147 0.232257 0.232257 0.232257 0.236802 0.236802 0.236802 0.243482 0.243482 0.243482 0.25 0.25 0.25 0.352841 0.352841 0.352841 0.352841
  line L6 (-8.75, 39.65) -> (33.15, 39.65)
  spline S7 degree 3 poles (39.65, 3) (39.65, 13.05) (39.65, 23.1) (39.65, 33.15) (39.65, 33.8012) (39.546, 34.6209) (39.2225, 35.4683) (38.9818, 36.0987) (38.6252, 36.7287) (38.1591, 37.2923) (37.4716, 38.1237) (36.5691, 38.7692) (35.6379, 39.155) (34.7327, 39.5301) (33.8456, 39.65) (33.15, 39.65) knots 0.873307 0.873307 0.873307 0.873307 0.976147 0.976147 0.976147 0.982257 0.982257 0.982257 0.986802 0.986802 0.986802 0.993482 0.993482 0.993482 1 1 1 1
  line L7 (39.65, 3) -> (39.65, -3)
  spline S8 degree 3 poles (8.75, -39.65) (16.8833, -39.65) (25.0167, -39.65) (33.15, -39.65) (33.8012, -39.65) (34.6209, -39.546) (35.4683, -39.2225) (36.0987, -38.9819) (36.7287, -38.6252) (37.2923, -38.1591) (38.1237, -37.4716) (38.7692, -36.5691) (39.155, -35.6379) (39.5301, -34.7327) (39.65, -33.8456) (39.65, -33.15) (39.65, -23.1) (39.65, -13.05) (39.65, -3) knots 0.64292 0.64292 0.64292 0.64292 0.726147 0.726147 0.726147 0.732257 0.732257 0.732257 0.736802 0.736802 0.736802 0.743482 0.743482 0.743482 0.75 0.75 0.75 0.852841 0.852841 0.852841 0.852841
extrude "Extrude12" cut sketch "Sketch20" against normal up to surface (8 mm away) contours L4 S5 L5 S6 L6 S7 L7 S8 bodies 4 in component "case"
component "switchesPlate" placed x (1, 0, 0) y (0, 1, 0) z (0, 0, 1) at (40.3063, -4.8609, 0.0689)
component "case" placed x (1, 0, 0) y (0, 1, 0) z (0, 0, 1) at (40.3063, -4.8609, 0.0689)
component "picoHolder" placed x (1, 0, 0) y (0, 1, 0) z (0, 0, 1) at (0, 0, 0)
hidden bodies 2
equation "d135 = 1\""
equation "d181 = d180"
equation "d182 = d180"
equation "d183 = d180"
equation "d208 = toleranceAdjust"
equation "d211 = toleranceAdjust"
equation "d246 = ( 51 / 2 ) * 1 mm"
equation "d247 = 21 mm / 2"
equation "toleranceAdjust = -0.5 mm"
equation "d261 = -toleranceAdjust"
named bodies: "switchPlate", "caseShellCutOut", "caseTop", "band", "caseBottom"
